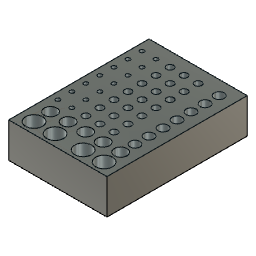
Bolt-Paint v3 (Autodesk Fusion 360 design; units mm, degrees)
Autodesk Fusion 360 part; units mm, degrees
sketch "Sketch1" plane through (0, 0, 0) normal (0, 0, 1) x (1, 0, 0)
  line L0 (-45, 50) -> (25, 50)
  line L1 (25, 50) -> (25, -50)
  line L2 (25, -50) -> (-45, -50)
  line L3 (-45, -50) -> (-45, 50)
  dimension "d1" = 70
  dimension "d2" = 100
  constraint horizontal L0
  constraint vertical L1
  constraint horizontal L2
  constraint vertical L3
  measures "d1" distance of L0.start L0.end
  measures "d2" distance of L0.start L2.end
extrude "Extrude1" add sketch "Sketch1" along normal blind 40
sketch "Sketch2" plane through (0, 0, 40) normal (0, 0, 1) x (-1, 0, 0)
  line L0 (45, 50) -> (-25, 50)
  line L1 (-25, 50) -> (-25, -50)
  line L2 (-25, -50) -> (45, -50)
  line L3 (45, -50) -> (45, 50)
  line L4 (40, -50) -> (40, 50) construction
  line L5 (30, -50) -> (30, 50) construction
  line L6 (20, -50) -> (20, 50) construction
  line L7 (10, -50) -> (10, 50) construction
  line L8 (0, -50) -> (0, 50) construction
  line L9 (-15, -50) -> (-15, 50) construction
  line L10 (45, -40) -> (-25, -40) construction
  line L11 (45, -30) -> (-25, -30) construction
  line L12 (45, -20) -> (-25, -20) construction
  line L13 (45, -10) -> (-25, -10) construction
  line L14 (45, 35) -> (-25, 35) construction
  line L15 (45, 45) -> (-25, 45) construction
  circle A0 centre (40, -40) radius 1.5
  circle A1 centre (40, -30) radius 1.5
  circle A2 centre (40, -20) radius 1.5
  circle A3 centre (40, -10) radius 1.5
  line L16 (45, 0) -> (-25, 0) construction
  line L17 (45, 10) -> (-25, 10) construction
  line L18 (45, 20) -> (-25, 20) construction
  line L19 (45, 30) -> (-25, 30) construction
  line L20 (-25, 42) -> (45, 42) construction
  circle A4 centre (40, 0) radius 1.5 construction
  circle A5 centre (40, 0) radius 1.5
  circle A6 centre (40, 10) radius 1.5
  circle A7 centre (40, 20) radius 1.5
  circle A8 centre (30, 0) radius 1.5
  circle A9 centre (30, -30) radius 1.5
  circle A10 centre (30, 20) radius 1.5
  circle A11 centre (30, 0) radius 1.5 construction
  circle A12 centre (30, -40) radius 1.5
  circle A13 centre (30, -20) radius 1.5
  circle A14 centre (30, 10) radius 1.5
  circle A15 centre (30, -10) radius 1.5
  circle A16 centre (0, -40) radius 2.5
  circle A17 centre (0, -30) radius 2.5
  circle A18 centre (0, -20) radius 2.5
  circle A19 centre (0, -10) radius 2.5
  circle A20 centre (0, 10) radius 2.5
  circle A21 centre (0, 0) radius 2.5
  circle A22 centre (0, 10) radius 2.5
  circle A23 centre (0, 20) radius 2.5
  circle A24 centre (10, 0) radius 2.5
  circle A25 centre (10, 10) radius 2.5
  circle A26 centre (10, 20) radius 2.5
  circle A27 centre (10, 10) radius 2.5
  circle A28 centre (10, -40) radius 2.5
  circle A29 centre (10, -20) radius 2.5
  circle A30 centre (10, -10) radius 2.5
  circle A31 centre (10, -30) radius 2.5
  circle A32 centre (20, 0) radius 2.5
  circle A33 centre (20, 10) radius 2.5
  circle A34 centre (20, 20) radius 2.5
  circle A35 centre (20, 10) radius 2.5
  circle A36 centre (20, -40) radius 2.5
  circle A37 centre (20, -20) radius 2.5
  circle A38 centre (20, -10) radius 2.5
  circle A39 centre (20, -30) radius 2.5
  circle A40 centre (-15, -40) radius 3.5
  circle A41 centre (-15, -30) radius 3.5
  circle A42 centre (-15, -20) radius 3.5
  circle A43 centre (-15, 0) radius 3.5
  circle A44 centre (-15, -10) radius 3.5
  circle A45 centre (-15, 10) radius 3.5
  circle A46 centre (-15, 20) radius 3.5
  circle A47 centre (35.1971, 30) radius 4.5
  circle A48 centre (10.1971, 30) radius 4.5
  circle A49 centre (-14.8029, 30) radius 4.5
  circle A50 centre (35, 42) radius 6
  circle A51 centre (0, 42) radius 6
  circle A52 centre (20, 42) radius 6
  circle A53 centre (-15, 42) radius 6
  circle A54 centre (35.1971, 30) radius 4.5
  circle A55 centre (22.6971, 30) radius 4.5
  circle A56 centre (-2.3029, 30) radius 4.5
  point P0 (10, -50)
  point P1 (10, 0)
  point P2 (20, -50)
  point P3 (20, 0)
  point P4 (-15, -20)
  dimension "d5" = 3
  dimension "d6" = 3
  dimension "d7" = 3
  dimension "d8" = 3
  dimension "d9" = 3
  dimension "d10" = 3
  dimension "d11" = 3
  dimension "d12" = 3
  dimension "d13" = 3
  dimension "d14" = 3
  dimension "d15" = 3
  dimension "d16" = 3
  dimension "d17" = 3
  dimension "d18" = 3
  dimension "d19" = 3
  dimension "d20" = 3
  dimension "d39" = 5
  dimension "d40" = 5
  dimension "d41" = 5
  dimension "d42" = 5
  dimension "d43" = 5
  dimension "d44" = 5
  dimension "d45" = 5
  dimension "d46" = 5
  dimension "d47" = 5
  dimension "d48" = 5
  dimension "d49" = 5
  dimension "d50" = 5
  dimension "d51" = 5
  dimension "d52" = 5
  dimension "d53" = 5
  dimension "d54" = 5
  dimension "d55" = 5
  dimension "d56" = 5
  dimension "d57" = 5
  dimension "d58" = 5
  dimension "d59" = 5
  dimension "d60" = 5
  dimension "d61" = 5
  dimension "d62" = 5
  dimension "d63" = 7
  dimension "d64" = 7
  dimension "d65" = 7
  dimension "d66" = 7
  dimension "d67" = 7
  dimension "d68" = 7
  dimension "d69" = 7
  dimension "d70" = 9
  dimension "d71" = 9
  dimension "d72" = 9
  dimension "d73" = 12
  dimension "d74" = 12
  dimension "d75" = 12
  dimension "d76" = 12
  dimension "d77" = 9
  dimension "d78" = 9
  dimension "d79" = 9
  constraint coincident L2 L4.start
  constraint coincident L0 L4.end
  constraint perpendicular L0 L4
  constraint coincident L2 L5.start
  constraint coincident L0 L5.end
  constraint perpendicular L0 L5
  constraint coincident L2 P2
  constraint coincident L0 L6.end
  constraint perpendicular L0 L6
  constraint midpoint L0 L7.end
  constraint coincident L2 L8.start
  constraint coincident L0 L8.end
  constraint perpendicular L0 L8
  constraint coincident L2 L9.start
  constraint coincident L0 L9.end
  constraint perpendicular L0 L9
  constraint coincident L3 L10.start
  constraint coincident L1 L10.end
  constraint perpendicular L1 L10
  constraint coincident L3 L11.start
  constraint coincident L1 L11.end
  constraint perpendicular L1 L11
  constraint coincident L3 L12.start
  constraint coincident L1 L12.end
  constraint perpendicular L1 L12
  constraint coincident L3 L13.start
  constraint coincident L1 L13.end
  constraint perpendicular L1 L13
  constraint coincident L3 L14.start
  constraint coincident L1 L14.end
  constraint perpendicular L1 L14
  constraint coincident L3 L15.start
  constraint coincident L1 L15.end
  constraint perpendicular L1 L15
  constraint coincident L10 A0.centre
  constraint coincident L4 A0.centre
  constraint coincident L4 A1.centre
  constraint coincident L11 A1.centre
  constraint coincident L4 A2.centre
  constraint coincident L12 A2.centre
  constraint coincident L4 A3.centre
  constraint coincident L13 A3.centre
  constraint midpoint L3 L16.start
  constraint midpoint L1 L16.end
  constraint coincident L3 L17.start
  constraint coincident L1 L17.end
  constraint perpendicular L1 L17
  constraint coincident L3 L18.start
  constraint coincident L1 L18.end
  constraint perpendicular L1 L18
  constraint coincident L3 L19.start
  constraint coincident L1 L19.end
  constraint perpendicular L1 L19
  constraint coincident L1 L20.start
  constraint coincident L3 L20.end
  constraint perpendicular L3 L20
  constraint midpoint L4 A4.centre
  constraint concentric A4 A5
  constraint coincident L4 A6.centre
  constraint coincident L17 A6.centre
  constraint coincident L4 A7.centre
  constraint coincident L18 A7.centre
  constraint concentric A8 A11
  constraint coincident L10 A16.centre
  constraint coincident L8 A16.centre
  constraint coincident L10 A40.centre
  constraint coincident L19 A47.centre
  constraint coincident L20 A50.centre
  measures "d5" diameter of A0
  measures "d6" diameter of A1
  measures "d7" diameter of A2
  measures "d8" diameter of A3
  measures "d9" diameter of A4
  measures "d10" diameter of A5
  measures "d11" diameter of A6
  measures "d12" diameter of A7
  measures "d13" diameter of A12
  measures "d14" diameter of A9
  measures "d15" diameter of A13
  measures "d16" diameter of A15
  measures "d17" diameter of A11
  measures "d18" diameter of A8
  measures "d19" diameter of A14
  measures "d20" diameter of A10
  measures "d39" diameter of A16
  measures "d40" diameter of A17
  measures "d41" diameter of A18
  measures "d42" diameter of A19
  measures "d43" diameter of A20
  measures "d44" diameter of A21
  measures "d45" diameter of A22
  measures "d46" diameter of A23
  measures "d47" diameter of A28
  measures "d48" diameter of A31
  measures "d49" diameter of A29
  measures "d50" diameter of A30
  measures "d51" diameter of A27
  measures "d52" diameter of A24
  measures "d53" diameter of A25
  measures "d54" diameter of A26
  measures "d55" diameter of A36
  measures "d56" diameter of A39
  measures "d57" diameter of A37
  measures "d58" diameter of A38
  measures "d59" diameter of A35
  measures "d60" diameter of A32
  measures "d61" diameter of A33
  measures "d62" diameter of A34
  measures "d63" diameter of A40
  measures "d64" diameter of A41
  measures "d65" diameter of A42
  measures "d66" diameter of A44
  measures "d67" diameter of A43
  measures "d68" diameter of A45
  measures "d69" diameter of A46
  measures "d70" diameter of A47
  measures "d71" diameter of A48
  measures "d72" diameter of A49
  measures "d73" diameter of A50
  measures "d74" diameter of A51
  measures "d75" diameter of A52
  measures "d76" diameter of A53
  measures "d77" diameter of A54
  measures "d78" diameter of A55
  measures "d79" diameter of A56
extrude "Extrude2" add sketch "Sketch2" along normal blind 20
sketch "Sketch3" plane through (0, 0, 60) normal (0, 0, 1) x (-1, 0, 0)
  circle A0 centre (-2.3029, 30) radius 4.5
  circle A1 centre (35.1971, 30) radius 4.5
  circle A2 centre (22.6971, 30) radius 4.5
  circle A3 centre (20, 42) radius 6
  circle A4 centre (0, 42) radius 6
  circle A5 centre (-15, 42) radius 6
  circle A6 centre (-15, 10) radius 3.5
  circle A7 centre (-14.8029, 30) radius 4.5
  circle A8 centre (35, 42) radius 6
  circle A9 centre (10, -40) radius 2.5
  circle A10 centre (30, -20) radius 1.5
  circle A11 centre (30, 10) radius 1.5
  circle A12 centre (30, -10) radius 1.5
  circle A13 centre (0, -40) radius 2.5
  circle A14 centre (0, -30) radius 2.5
  circle A15 centre (0, -20) radius 2.5
  circle A16 centre (0, -10) radius 2.5
  circle A17 centre (0, 0) radius 2.5
  circle A18 centre (0, 20) radius 2.5
  circle A19 centre (10, -30) radius 2.5
  circle A20 centre (20, 0) radius 2.5
  circle A21 centre (10, 20) radius 2.5
  circle A22 centre (10, 0) radius 2.5
  circle A23 centre (0, 10) radius 2.5
  circle A24 centre (10, -20) radius 2.5
  circle A25 centre (10, -10) radius 2.5
  circle A26 centre (-15, -10) radius 3.5
  circle A27 centre (30, -40) radius 1.5
  circle A28 centre (20, 20) radius 2.5
  circle A29 centre (40, 20) radius 1.5
  circle A30 centre (20, 10) radius 2.5
  circle A31 centre (30, 20) radius 1.5
  circle A32 centre (-15, -20) radius 3.5
  circle A33 centre (40, -20) radius 1.5
  circle A34 centre (40, -40) radius 1.5
  circle A35 centre (30, -30) radius 1.5
  circle A36 centre (-15, 0) radius 3.5
  circle A37 centre (10, 10) radius 2.5
  circle A38 centre (30, 0) radius 1.5
  circle A39 centre (20, -30) radius 2.5
  circle A40 centre (-15, -30) radius 3.5
  circle A41 centre (40, 10) radius 1.5
  circle A42 centre (40, -10) radius 1.5
  circle A43 centre (40, 0) radius 1.5
  circle A44 centre (20, -40) radius 2.5
  circle A45 centre (20, -20) radius 2.5
  circle A46 centre (40, -30) radius 1.5
  circle A47 centre (-15, -40) radius 3.5
  circle A48 centre (20, -10) radius 2.5
  circle A49 centre (-15, 20) radius 3.5
  circle A50 centre (10.1971, 30) radius 4.5
  line L0 (45, -50) -> (45, 50)
  line L1 (45, 50) -> (-25, 50)
  line L2 (-25, 50) -> (-25, -50)
  line L3 (-25, -50) -> (45, -50)
extrude "Extrude3" cut 1 faces at (-21.6667, 16.6667, 0) along direction (0, 0, 1) blind 15
sketch "Sketch4" plane through (0, 0, 15) normal (0, 0, -1) x (1, 0, 0)
  line L0 (25, 50) -> (-45, 50)
  line L1 (-45, 50) -> (-45, -50)
  line L2 (-45, -50) -> (25, -50)
  line L3 (25, -50) -> (25, 50)
  line L4 (-25, -50) -> (-45, -50)
  line L5 (-45, -50) -> (-45, 15)
  line L6 (-45, 15) -> (-25, 15)
  line L7 (-25, 15) -> (-25, -50)
  constraint horizontal L4
  constraint vertical L5
  constraint horizontal L6
  constraint vertical L7
  constraint coincident L1 L5.end
  constraint coincident L2 L4.start
extrude "Extrude4" add sketch "Sketch4" against normal blind 35 contours L1 L2 L4 L5 L6 L7
sketch "Sketch5" plane through (0, 0, 15) normal (0, 0, -1) x (1, 0, 0)
  line L0 (-45, -50) -> (25, -50)
  line L1 (25, -50) -> (25, 50)
  line L2 (25, 50) -> (-45, 50)
  line L3 (-45, 50) -> (-45, -50)
  line L4 (-25, -50) -> (-25, -70)
  line L5 (-25, -70) -> (-15, -75)
  line L6 (5, -50) -> (5, -65)
  line L7 (-45, 23.0126) -> (-75, 23.0126)
  line L8 (5, -50) -> (-25, -50)
  line L9 (-25, -50) -> (-25, 23.0126)
  line L10 (-25, 23.0126) -> (5, 23.0126)
  line L11 (5, 23.0126) -> (5, -50)
  dimension "d86" = 11.1803
  constraint coincident L0 L4.start
  constraint perpendicular L0 L4
  constraint coincident L0 L6.start
  constraint perpendicular L0 L6
  constraint coincident L3 L7.start
  constraint perpendicular L3 L7
  constraint horizontal L8
  constraint vertical L9
  constraint horizontal L10
  constraint vertical L11
  measures "d86" distance of L4.end L5.end
extrude "Extrude5" add sketch "Sketch5" against normal blind 25 contours L0 L8 L9 L10 L11
extrude "Extrude6" cut 1 faces at (1.6667, 16.6667, 15) along direction (0, 0, 1) blind 20
